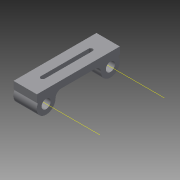
# Autodesk Inventor part: Sensor stand
Saved by Autodesk Inventor 2013 (Build 170138000, 138)
## iProperties
Created: 2013-01-04
Part Number: Sensor stand
Material: Generic
Document SubType Name: Modeling
Designer: Nico
Density: 1 g/cm^3
Author: Nico
Autodesk Inventor part; units mm, degrees
ref_plane "YZ Plane" through (0, 0, 0) normal (1, 0, 0) x (0, 1, 0)
ref_plane "XZ Plane" through (0, 0, 0) normal (0, 1, 0) x (-1, 0, 0)
ref_plane "XY Plane" through (0, 0, 0) normal (0, 0, 1) x (1, 0, 0)
sketch "Sketch1" plane through (0, 0, 0) normal (0, 0, 1) x (1, 0, 0)
  line L0 (0, 0) -> (20, 0)
  line L1 (20, 0) -> (20, 71)
  line L2 (20, 71) -> (0, 71)
  line L3 (0, 71) -> (0, 0)
  dimension "d0" = 20
  dimension "d1" = 71
  constraints: 8 end point, 2 parallel, 1 horizontal, 1 perpendicular
  measures "d0" distance of L0.start L0.end
  measures "d1" distance of L2.end L0.start
extrude "Extrusion1" add sketch "Sketch1" along normal blind 6
sketch "Sketch3" plane through (20, 0, 0) normal (1, 0, 0) x (0, 0, -1)
  line L0 (0, 0) -> (0, 71) projected
  circle A0 centre (5, 62.9091) radius 3.9
  circle A1 centre (5, 7.9091) radius 3.9
  circle A2 centre (5, 62.9091) radius 8
  circle A3 centre (5, 7.9091) radius 8
  dimension "d19" = 7.8
  dimension "d21" = 7.8
  dimension "d22" = 55
  dimension "d24" = 16
  dimension "d25" = 16
  dimension "d26" = 5
  dimension "d31" = 5
  constraints: 4 centre point, 2 coincident
  measures "d19" diameter of A0
  measures "d21" diameter of A1
  measures "d22" distance of A1.centre A0.centre
  measures "d24" diameter of A2
  measures "d25" diameter of A3
  measures "d26" distance from line of A0.centre L0
  measures "d31" distance from line of L0 A1.centre
extrude "Extrusion3" add sketch "Sketch3" against normal blind 20
fillet "Fillet1" radius 1 1 edges at (10, 69.1541, 0)
fillet "Fillet2" radius 1 1 edges at (10, 1.6641, 0)
fillet "Fillet3" radius 5 2 edges at (10, 56.6641, 0) (10, 14.1541, 0)
sketch "Sketch4" plane through (0, 0, 6) normal (0, 0, 1) x (1, 0, 0)
  line L0 (0, 0) -> (20, 0) projected
  line L1 (20, 71) -> (0, 71) projected
  circle A0 centre (10, 56) radius 1.75
  circle A1 centre (10, 15) radius 1.75
  line L2 (8.25, 56) -> (11.75, 56)
  line L3 (11.75, 56) -> (11.75, 15)
  line L4 (11.75, 15) -> (8.25, 15)
  line L5 (8.25, 15) -> (8.25, 56)
  dimension "d42" = 3.5
  dimension "d43" = 3.5
  dimension "d40" = 15
  dimension "d41" = 15
  constraints: 8 end point, 2 horizontal alignment, 2 parallel, 1 horizontal, 1 perpendicular, 4 other
  measures "d40" distance from line of L1 point (10, 56)
  measures "d41" distance from line of L0 point (10, 15)
extrude "Extrusion4" cut sketch "Sketch4" against normal blind 10
body "Solid1"
